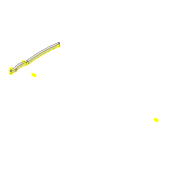
# Autodesk Inventor part: Part_9
Saved by Autodesk Inventor 2022 (Build 260153000, 153)
## iProperties
Created: 2022-04-26
Part Number: Part_9
Material: Generic
Document SubType Name: Modeling
Designer: dell
Density: 1 g/cm^3
Appearance: Default
Author: dell
Autodesk Inventor part; units mm, degrees
ref_plane "YZ Plane" through (0, 0, 0) normal (1, 0, 0) x (0, 1, 0)
ref_plane "XZ Plane" through (0, 0, 0) normal (0, 1, 0) x (-1, 0, 0)
ref_plane "XY Plane" through (0, 0, 0) normal (0, 0, 1) x (1, 0, 0)
sketch "Sketch1" plane through (0, 0, 0) normal (0, 1, 0) x (-1, 0, 0)
  line L0 (0, 0) -> (0, -167.039) construction
  line L1 (-3, 0) -> (-3, -167.039)
  line L2 (3, -167.039) -> (3, 0)
  arc A0 (3, 0) -> (-3, 0) centre (0, 0) ccw
  arc A1 (-3, -167.039) -> (3, -167.039) centre (0, -167.039) ccw
  circle A2 centre (0, 0) radius 1.5
  circle A3 centre (0, -167.039) radius 1.5
  circle A4 centre (0, -57.227) radius 1.5
  arc A5 (3, -167.039) -> (3, -57.227) centre (-393.2137, -112.133) ccw
  arc A6 (-3, -167.039) -> (-3, -57.227) centre (-399.2137, -112.133) ccw
  arc A7 (-3, -55) -> (-3, -15) centre (-48.8258, -35) ccw
  arc A8 (3, -55) -> (3, -15) centre (-42.8258, -35) ccw
  point P0 (0, -83.5195)
  dimension "d0" = 167.039
  dimension "d1" = 6
  dimension "d2" = 3
  dimension "d3" = 3
  dimension "d10" = 3
  dimension "d11" = 57.227
  dimension "d12" = 400
  dimension "d13" = 400
  dimension "d16" = 15
  dimension "d17" = 55
  dimension "d18" = 50
  dimension "d19" = 50
  constraints: 12 point on circle, 9 centre point, 9 point on line, 8 end point, 6 horizontal alignment, 4 tangent, 2 coincident, 1 midpoint, 1 parallel, 1 vertical
  measures "d0" distance of L0.start L0.end
  measures "d1" diameter of A1
  measures "d2" diameter of A2
  measures "d3" diameter of A3
  measures "d10" diameter of A4
  measures "d11" distance of L0.start A4.centre
  measures "d12" radius of A6
  measures "d13" radius of A5
  measures "d16" vertical distance of A7.end L0.start
  measures "d17" vertical distance of A7.start L0.start
  measures "d18" radius of A7
  measures "d19" radius of A8
extrude "Extrusion1" add sketch "Sketch1" along normal blind 8 contours A0 L2 A1 A6 L1 A7 | A8 L2 | A5 L2
fillet "Fillet1" radius 10 6 edges at (-3, 4, -15) (3, 4, -15) (-3, 4, -55) (3, 4, -55) (-3, 4, -57.227) (3, 4, -57.227)
sketch "Sketch2" plane through (0, 0, 0) normal (0, -1, 0) x (1, 0, 0)
  circle A0 centre (0, -57.227) radius 1.5 projected
  circle A1 centre (0, -167.039) radius 1.5 projected
  circle A2 centre (0, 0) radius 1.5 projected
  arc A3 (2.8635, -58.2209) -> (2.2666, -53.2276) centre (-7.0452, -56.8731) ccw projected
  arc A4 (2.3043, -16.6764) -> (2.2666, -53.2276) centre (48.8258, -35) ccw projected
  arc A5 (2.3043, -16.6764) -> (3, -13.0117) centre (-7, -13.0117) ccw projected
  line L0 (3, 0) -> (3, -13.0117) projected
  arc A6 (3, 0) -> (-3, 0) centre (0, 0) ccw projected
  line L1 (-3, -13.0117) -> (-3, 0) projected
  arc A7 (-3.6957, -16.6764) -> (-3, -13.0117) centre (-13, -13.0117) ccw projected
  arc A8 (-3.6957, -16.6764) -> (-3.7334, -53.2276) centre (42.8258, -35) ccw projected
  arc A9 (-3.1365, -58.2209) -> (-3.7334, -53.2276) centre (-13.0452, -56.8731) ccw projected
  arc A10 (-3.1365, -58.2209) -> (-3, -167.039) centre (393.2137, -112.133) ccw projected
  arc A11 (-3, -167.039) -> (3, -167.039) centre (0, -167.039) ccw projected
  arc A12 (2.8635, -58.2209) -> (3, -167.039) centre (399.2137, -112.133) ccw projected
body "Solid1"
